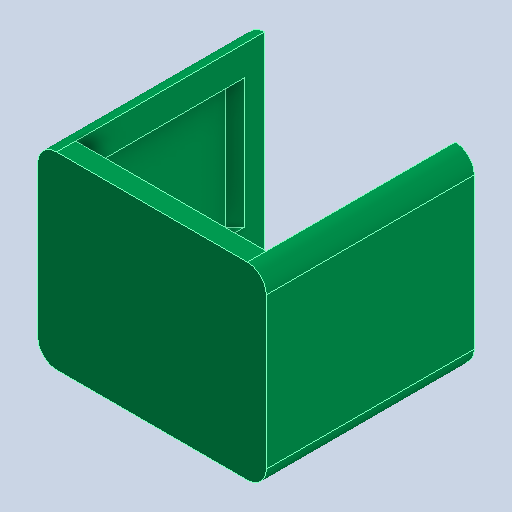
# Autodesk Inventor part: Cover Top (Full)
Saved by Autodesk Inventor 2023.1 (Build 271208000, 208)
## iProperties
Created: 2022-11-14
Part Number: Cover Top (Full)
Material: Generic
Document SubType Name: Modeling
Designer: xSibe
Density: 1 g/cm^3
Appearance: Plastic Dark Green
Author: xSibe
Autodesk Inventor part; units mm, degrees
ref_plane "YZ Plane" through (0, 0, 0) normal (1, 0, 0) x (0, 1, 0)
sketch "Sketch1" plane through (0, 0, 0) normal (0, 0, 1) x (1, 0, 0)
  circle A0 centre (-21.9, -21.9) radius 1.875 projected
  circle A1 centre (21.9, 21.9) radius 1.875 projected
  circle A2 centre (21.9, -21.9) radius 1.875 projected
  circle A3 centre (-21.9, 21.9) radius 1.875 projected
  circle A4 centre (14.4, 20.8) radius 2.0734 projected
  circle A5 centre (-14.4, -20.8) radius 2.0734 projected
  circle A6 centre (14.4, -20.8) radius 2.0734 projected
  circle A7 centre (20.8, -14.4) radius 2.0734 projected
  line L0 (-17.05, 17.05) -> (-17.05, -17.05) projected
  line L1 (17.05, 17.05) -> (-17.05, 17.05) projected
  line L2 (17.05, -17.05) -> (17.05, 17.05) projected
  line L3 (-17.05, -17.05) -> (17.05, -17.05) projected
  circle A8 centre (20.8, 14.4) radius 2.0734 projected
  circle A9 centre (-14.4, 20.8) radius 2.0734 projected
  circle A10 centre (-20.8, -14.4) radius 2.0734 projected
  circle A11 centre (-20.8, 14.4) radius 2.0734 projected
  line L4 (-22.9, 24.875) -> (22.9, 24.875) projected
  arc A12 (-22.9, 24.875) -> (-24.875, 22.9) centre (-22.9, 22.9) ccw projected
  line L5 (-24.875, -22.9) -> (-24.875, 22.9) projected
  arc A13 (-24.875, -22.9) -> (-22.9, -24.875) centre (-22.9, -22.9) ccw projected
  line L6 (22.9, -24.875) -> (-22.9, -24.875) projected
  arc A14 (22.9, -24.875) -> (24.875, -22.9) centre (22.9, -22.9) ccw projected
  line L7 (24.875, 22.9) -> (24.875, -22.9) projected
  arc A15 (24.875, 22.9) -> (22.9, 24.875) centre (22.9, 22.9) ccw projected
  line L8 (-24.875, 24.875) -> (24.875, 24.875)
  line L9 (24.875, 24.875) -> (24.875, -24.875)
  line L10 (24.875, -24.875) -> (-24.875, -24.875)
  line L11 (-24.875, -24.875) -> (-24.875, 24.875)
  line L12 (-24.875, 24.875) -> (24.875, -24.875) construction
  line L13 (24.875, 24.875) -> (-24.875, -24.875) construction
  point P0 (0, 0)
  constraints: 12 end point, 2 midpoint, 2 parallel, 2 tangent, 1 horizontal, 1 perpendicular
ref_plane "Work Plane1" through (-24.875, -24.875, 49.8) normal (0, 0, 1) x (1, 0, 0)
extrude "Extrusion1" add sketch "Sketch1" along normal blind 5 from surface at 49.8 contours A0 | A1 | A2 | A3 | A4 | A5 | A6 | A7 | L1 L2 L3 L0 | A8 | A9 | A10 | A11 | L4 A15 L7 A14 L6 A13 L5 A12 | A12 L11 L8 | L8 L9 A15 | A13 L10 L11 | L9 L10 A14
sketch "Sketch2" plane through (-24.875, 24.875, 54.8) normal (0, 0, 1) x (1, 0, 0)
  line L0 (49.75, 0) -> (49.75, -49.75) projected
  line L1 (0, 0) -> (49.75, 0) projected
  line L2 (0, -49.75) -> (0, 0) projected
  line L3 (49.75, -49.75) -> (0, -49.75) projected
  line L4 (49.75, -49.75) -> (50, -49.75)
  line L5 (50, -49.75) -> (50, 0)
  line L6 (50, 0) -> (49.75, 0)
  line L7 (49.75, 0) -> (49.75, -49.75)
  line L8 (50, -49.75) -> (55, -49.75)
  line L9 (55, -49.75) -> (55, 0)
  line L10 (55, 0) -> (50, 0)
  line L11 (50, 0) -> (50, -49.75)
  line L12 (24.875, -49.75) -> (24.875, 0)
  line L13 (0, 0) -> (0, -49.75)
  line L14 (0, -49.75) -> (-0.25, -49.75)
  line L15 (-0.25, -49.75) -> (-0.25, 0)
  line L16 (-0.25, 0) -> (0, 0)
  line L17 (0, 0) -> (0, -49.75)
  line L18 (-0.25, -49.75) -> (-5.25, -49.75)
  line L19 (-5.25, -49.75) -> (-5.25, 0)
  line L20 (-5.25, 0) -> (-0.25, 0)
  line L21 (-0.25, 0) -> (-0.25, -49.75)
  point P0 (24.875, -24.875)
  point P1 (-0.25, 0)
  point P2 (50, 0)
  point P3 (50, 0)
  point P4 (-0.25, 0)
  dimension "d2" = 0.25
  dimension "d3" = 49.75
  dimension "d4" = 5
  dimension "d5" = 49.75
  constraints: 36 end point, 7 symmetric about line, 4 parallel, 2 horizontal, 2 midpoint, 2 perpendicular
  measures "d2" distance of L6.end L5.end
  measures "d3" distance of L5.end L4.end
  measures "d4" distance of L10.end L9.end
  measures "d5" distance of L8.end L9.end
extrude "Extrusion2" add sketch "Sketch2" against normal blind 5 contours L6 L5 L4 L0 | L10 L9 L8 L5 | L2 L14 L15 L16 | L15 L18 L19 L20
ref_plane "Work Plane2" through (-24.875, -24.875, 0) normal (0, 0, -1) x (0, 1, 0)
extrude "Extrusion3" add sketch "Sketch2" against normal up to surface (54.8 mm away) contours L10 L9 L8 L5 | L15 L18 L19 L20
sketch "Sketch3" plane through (25.125, -24.875, 49.8) normal (-1, 0, 0) x (0, 0, 1)
  line L0 (-7.7, 7.825) -> (-42.1, 7.825) projected
  line L1 (-42.1, 41.925) -> (-7.7, 41.925) projected
  line L2 (-24.9, 7.825) -> (-24.9, 41.925)
  line L3 (-42.1, 7.825) -> (-7.7, 7.825)
  line L4 (-7.7, 7.825) -> (-7.7, 41.925)
  line L5 (-7.7, 41.925) -> (-42.1, 41.925)
  line L6 (-42.1, 41.925) -> (-42.1, 7.825)
  line L7 (-42.1, 7.825) -> (-7.7, 41.925) construction
  line L8 (-7.7, 7.825) -> (-42.1, 41.925) construction
  point P0 (-49.8, 24.875)
  point P1 (-24.9, 24.875)
  constraints: 14 end point, 5 midpoint, 2 parallel, 1 horizontal, 1 perpendicular
extrude "Extrusion4" cut sketch "Sketch3" against normal blind 2.5
mirror "Mirror1" about plane through (0, 0, 0) normal (1, 0, 0) of "Extrusion4"
sketch "Sketch4" plane through (25.125, -24.875, 49.8) normal (0, 0, -1) x (-1, 0, 0)
  circle A0 centre (47.025, 2.975) radius 1.875 projected
  circle A1 centre (3.225, 46.775) radius 1.875 projected
  circle A2 centre (3.225, 2.975) radius 1.875 projected
  circle A3 centre (47.025, 46.775) radius 1.875 projected
  circle A4 centre (10.725, 45.675) radius 2.0734 projected
  circle A5 centre (39.525, 4.075) radius 2.0734 projected
  circle A6 centre (10.725, 4.075) radius 2.0734 projected
  circle A7 centre (4.325, 10.475) radius 2.0734 projected
  line L0 (42.175, 41.925) -> (42.175, 7.825) projected
  line L1 (8.075, 41.925) -> (42.175, 41.925) projected
  line L2 (8.075, 7.825) -> (8.075, 41.925) projected
  line L3 (42.175, 7.825) -> (8.075, 7.825) projected
  circle A8 centre (4.325, 39.275) radius 2.0734 projected
  circle A9 centre (39.525, 45.675) radius 2.0734 projected
  circle A10 centre (45.925, 10.475) radius 2.0734 projected
  circle A11 centre (45.925, 39.275) radius 2.0734 projected
  line L4 (48.025, 49.75) -> (2.225, 49.75) projected
  arc A12 (50, 47.775) -> (48.025, 49.75) centre (48.025, 47.775) ccw projected
  line L5 (50, 1.975) -> (50, 47.775) projected
  arc A13 (48.025, 0) -> (50, 1.975) centre (48.025, 1.975) ccw projected
  line L6 (2.225, 0) -> (48.025, 0) projected
  arc A14 (0.25, 1.975) -> (2.225, 0) centre (2.225, 1.975) ccw projected
  line L7 (0.25, 47.775) -> (0.25, 1.975) projected
  arc A15 (2.225, 49.75) -> (0.25, 47.775) centre (2.225, 47.775) ccw projected
  point P0 (25.125, 24.875)
extrude "Extrusion5" cut sketch "Sketch4" against normal blind 2.5 contours A4 | A5 | A6 | L0 L3 L2 L1 | A9
chamfer "Chamfer1" distance 2.5 angle 45 8 edges at (-25.125, 0, 42.1) (-25.125, 0, 7.7) (25.125, 0, 42.1) (25.125, 0, 7.7) (0, 17.05, 49.8) (17.05, 0, 49.8) (-17.05, 0, 49.8) (0, -17.05, 49.8)
fillet "Fillet1" radius 5 4 edges at (30.125, -24.875, 27.4) (-30.125, -24.875, 27.4) (-30.125, 24.875, 27.4) (30.125, 24.875, 27.4)
body "Solid1"
